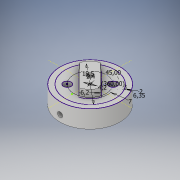
# Autodesk Inventor part: InputMountingHub
Saved by Autodesk Inventor 2018.3 (Build 223284000, 284)
## iProperties
Created: 2018-08-27
Part Number: InputMountingHub
Material: Generisch
Document SubType Name: Modeling
Designer: JochenAlt
Density: 1 g/cm^3
Appearance: Vorgabe
Author: JochenAlt
Autodesk Inventor part; units mm, degrees
ref_plane "YZ Plane" through (0, 0, 0) normal (1, 0, 0) x (0, 1, 0)
ref_plane "XZ Plane" through (0, 0, 0) normal (0, 1, 0) x (-1, 0, 0)
ref_plane "XY Plane" through (0, 0, 0) normal (0, 0, 1) x (1, 0, 0)
sketch "Skizze1" plane through (0, 0, 0) normal (0, 0, 1) x (1, 0, 0)
  circle A0 centre (0, 0) radius 9.75
  line L0 (0, 16.45) -> (0, -16.45) construction
  line L1 (-16.45, 0) -> (16.45, 0) construction
  circle A1 centre (4.490128, 4.490128) radius 1.5
  circle A2 centre (0, 0) radius 6.35 construction
  circle A3 centre (-4.490128, -4.490128) radius 1.5
  circle A4 centre (0, 0) radius 11.75
  line L2 (4.490128, 4.490128) -> (0, 0) construction
  circle A5 centre (0, 0) radius 2.1
  circle A6 centre (0, 0) radius 1.2
  arc A7 (2.245874, -6.629936) -> (6.629936, -2.245874) centre (0, 0) ccw
  line L3 (6.629936, -2.245874) -> (-2.245874, 6.629936)
  line L4 (-6.629936, 2.245874) -> (2.245874, -6.629936)
  arc A8 (-2.245874, 6.629936) -> (-6.629936, 2.245874) centre (0, 0) ccw
  arc A9 (-2.245874, 6.629936) -> (-6.629936, 2.245874) centre (0, 0) ccw
  line L5 (0, 0) -> (4.949747, -4.949747) construction
  point P0 (0, -7)
  dimension "d3" = 6.35
  dimension "d0" = 19.5
  dimension "d1" = 3
  dimension "d6" = 360
  dimension "d8" = 2
  dimension "d17" = 45
  dimension "d21" = 4.2
  dimension "d24" = 2.4
  dimension "d76" = 7
  dimension "d122" = 6.2
  constraints: 9 centre point, 8 coincident, 8 end point, 7 point on circle, 2 perpendicular, 1 concentric, 1 parallel, 1 point on line, 9 other
  measures "d0" diameter of A0
  measures "d1" diameter of A1
  measures "d8" radial gap between concentric circles of A4 A0
  measures "d17" angle of L0 L2
  measures "d21" diameter of A5
  measures "d24" diameter of A6
  measures "d76" radius of A7
  measures "d122" distance between parallel lines of L4 L3
extrude "Extrusion1" add sketch "Skizze1" against normal blind 7 contours A4
extrude "Extrusion2" add sketch "Skizze1" against normal blind 2 contours A0 | A4 | A5 | A6 | L4 A8 L3 A7
sketch "Skizze2" plane through (0, 0, 0) normal (0, 1, 0) x (-1, 0, 0)
  circle A0 centre (0, -4.5) radius 1
  line L0 (-9.75, 0) -> (9.75, 0) projected
  point P0 (0, 0)
  dimension "d13" = 2
  dimension "d14" = 4.5
  constraints: 1 centre point
  measures "d13" diameter of A0
  measures "d14" distance from line of A0.centre L0
extrude "Extrusion3" cut sketch "Skizze2" along normal through all both and the other way through all
sketch "Skizze1 outline for Extrusion4" plane through (0, 0, 0) normal (0, 0, 1) x (1, 0, 0)
  arc A0 (2.245874, -6.629936) -> (6.629936, -2.245874) centre (0, 0) ccw
  line L0 (-6.629936, 2.245874) -> (2.245874, -6.629936)
  arc A1 (-2.245874, 6.629936) -> (-6.629936, 2.245874) centre (0, 0) ccw
  line L1 (6.629936, -2.245874) -> (-2.245874, 6.629936)
extrude "Extrusion4" add sketch "Skizze1 outline for Extrusion4" along normal blind 3 draft -5
extrude "Extrusion6" cut sketch "Skizze1" along normal through all both and the other way through all contours A6
extrude "Extrusion7" cut sketch "Skizze1" along normal blind 2 from surface at -2 contours A5
